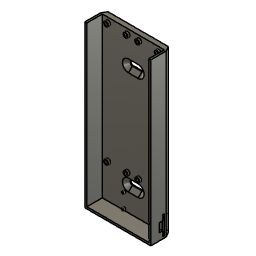
baseplate v1 (Autodesk Fusion 360 design; units mm, degrees)
Autodesk Fusion 360 part; units mm, degrees
sketch "Skizze1" plane through (0, 0, 0) normal (0, 0, 1) x (1, 0, 0)
  line L0 (0, 0) -> (62.5, 0)
  line L1 (62.5, 0) -> (62.5, 165)
  line L2 (62.5, 165) -> (0, 165)
  line L3 (0, 165) -> (0, 0)
  line L4 (31.25, 165) -> (31.25, 0) construction
  line L5 (0, 82.5) -> (62.5, 82.5) construction
  line L6 (57.5, 160) -> (5, 160) construction
  line L7 (5, 160) -> (5, 36) construction
  line L8 (5, 36) -> (57.5, 36) construction
  line L9 (57.5, 36) -> (57.5, 160) construction
  line L10 (57.5, 160) -> (5, 36) construction
  line L11 (5, 160) -> (57.5, 36) construction
  circle A0 centre (5, 36) radius 2.5
  circle A1 centre (57.5, 36) radius 2.5
  circle A2 centre (57.5, 160) radius 2.5
  circle A3 centre (5, 160) radius 2.5
  line L12 (22.1877, 17.0911) -> (63.1877, 17.0911) construction
  line L13 (63.1877, 17.0911) -> (63.1877, 2.0911) construction
  line L14 (63.1877, 2.0911) -> (22.1877, 2.0911) construction
  line L15 (22.1877, 2.0911) -> (22.1877, 17.0911) construction
  circle A4 centre (63.1877, 17.0911) radius 1.25
  circle A5 centre (63.1877, 2.0911) radius 1.25
  circle A6 centre (22.1877, 17.0911) radius 1.25
  circle A7 centre (22.1877, 2.0911) radius 1.25
  circle A8 centre (16.25, 26.2295) radius 6.25
  circle A9 centre (46.25, 26.2295) radius 6.25
  line L16 (0, 26.2295) -> (62.5, 26.2295) construction
  line L17 (37.25, 160) -> (25.25, 160) construction
  line L18 (25.25, 160) -> (25.25, 36) construction
  line L19 (25.25, 36) -> (37.25, 36) construction
  line L20 (37.25, 36) -> (37.25, 160) construction
  line L21 (37.25, 160) -> (25.25, 36) construction
  line L22 (25.25, 160) -> (37.25, 36) construction
  circle A10 centre (25.25, 160) radius 2.5
  circle A11 centre (37.25, 160) radius 2.5
  circle A12 centre (25.25, 36) radius 2.5
  circle A13 centre (37.25, 36) radius 2.5
  point P0 (31.25, 98)
  point P1 (31.25, 98)
  dimension "d1" = 62.5
  dimension "d2" = 165
  dimension "d3" = 52.5
  dimension "d4" = 124
  dimension "d5" = 5
  dimension "d6" = 5
  dimension "d7" = 5
  dimension "d8" = 5
  dimension "d9" = 5
  dimension "d10" = 41
  dimension "d11" = 15
  dimension "d13" = 2.5
  dimension "d14" = 2.5
  dimension "d15" = 2.5
  dimension "d16" = 2.5
  dimension "d17" = 12.5
  dimension "d18" = 12.5
  dimension "d19" = 15
  dimension "d20" = 15
  dimension "d25" = 12
  dimension "d26" = 5
  dimension "d27" = 5
  dimension "d28" = 5
  dimension "d29" = 5
  dimension "d30" = 124
  constraint horizontal L0
  constraint vertical L1
  constraint horizontal L2
  constraint vertical L3
  constraint coincident L0.start L3.end
  constraint midpoint L2 L4.start
  constraint midpoint L0 L4.end
  constraint midpoint L3 L5.start
  constraint midpoint L1 L5.end
  constraint horizontal L6
  constraint perpendicular L6 L7
  constraint parallel L6 L8
  constraint parallel L7 L9
  constraint coincident L10 P1
  constraint coincident L11 P1
  constraint coincident L4 P1
  constraint coincident L7.end L8.start
  constraint coincident L8.end L9.start
  constraint coincident L6.start L9.end
  constraint coincident L6.end L7.start
  constraint horizontal L12
  constraint vertical L13
  constraint horizontal L14
  constraint vertical L15
  constraint coincident L12.end L13.start
  constraint coincident L13.end L14.start
  constraint coincident L12.start L15.end
  constraint coincident L14.end L15.start
  constraint coincident L3 L16.start
  constraint coincident L1 L16.end
  constraint perpendicular L1 L16
  constraint coincident A9.centre L16
  constraint coincident A8.centre L16
  constraint horizontal L17
  constraint perpendicular L17 L18
  constraint parallel L17 L19
  constraint parallel L18 L20
  constraint coincident L21 P1
  constraint coincident L22 P1
  constraint coincident P1 P0
  constraint coincident L17.end L18.start
  constraint coincident L17.start L20.end
  constraint coincident L18.end L19.start
  constraint coincident L19.end L20.start
  measures "d1" distance of L0.start L0.end
  measures "d2" distance of L0.start L2.end
  measures "d3" distance of L7.end L8.end
  measures "d4" distance of L6.end L7.end
  measures "d5" distance of L2 L6
  measures "d6" diameter of A0
  measures "d7" diameter of A1
  measures "d8" diameter of A2
  measures "d9" diameter of A3
  measures "d10" distance of L12.start L12.end
  measures "d11" distance of L12.start L14.end
  measures "d13" diameter of A4
  measures "d14" diameter of A5
  measures "d15" diameter of A6
  measures "d16" diameter of A7
  measures "d17" diameter of A8
  measures "d18" diameter of A9
  measures "d19" distance of L4 A8.centre
  measures "d20" distance of L4 A9.centre
  measures "d25" distance of L18.end L19.end
  measures "d26" diameter of A10
  measures "d27" diameter of A11
  measures "d28" diameter of A12
  measures "d29" diameter of A13
  measures "d30" distance of L17.end L18.end
extrude "Extrusion1" add sketch "Skizze1" along normal blind 5 contours L0 L1 L2 L3 A4 A5 | L1 A5 | L1 A4 | A0 | A1 | A2 | A3 | A6 | A7 | A8 | A9 | A10 | A11 | A12 | A13 picked at (62.3027, 2.2267) picked at (62.3167, 17.1498)
extrude "Extrusion2" add sketch "Skizze1" along normal blind 7 contours L1 A5 | L1 A5 | L1 A4 | L1 A4 | A0 | A1 | A2 | A3 | A6 | A7 | A10 | A11 | A12 | A13
hole "Bohrung1" at (5, 160, 7) direction (0, 0, -1) diameter 2.6 depth 5 tip angle 180
hole "Bohrung2" at (25.25, 160, 7) direction (0, 0, -1) diameter 2.6 depth 5 tip angle 180
hole "Bohrung3" at (37.25, 160, 7) direction (0, 0, -1) diameter 2.6 depth 5 tip angle 180
hole "Bohrung4" at (57.5, 160, 7) direction (0, 0, -1) diameter 2.6 depth 5 tip angle 180
hole "Bohrung5" at (5, 36, 7) direction (0, 0, -1) diameter 2.6 depth 5 tip angle 180
hole "Bohrung6" at (25.25, 36, 7) direction (0, 0, -1) diameter 2.6 depth 5 tip angle 180
hole "Bohrung7" at (37.25, 36, 7) direction (0, 0, -1) diameter 2.6 depth 5 tip angle 180
hole "Bohrung8" at (57.5, 36, 7) direction (0, 0, -1) diameter 2.6 depth 5 tip angle 180
hole "Bohrung9" at (22.1877, 17.0911, 7) direction (0, 0, -1) diameter 1 depth 5 tip angle 180
hole "Bohrung10" at (22.1877, 2.0911, 7) direction (0, 0, -1) diameter 1 depth 5 tip angle 180
sketch "Skizze2" plane through (0, 165, 0) normal (0, 1, 0) x (-1, 0, 0)
  line L0 (-62.5, 0) -> (0, 0)
  line L1 (0, 0) -> (0, 5)
  line L2 (0, 5) -> (-62.5, 5)
  line L3 (-62.5, 5) -> (-62.5, 0)
  line L4 (0, 0) -> (2.8868, 5)
  line L5 (0, 0) -> (5.7735, 0) construction
  line L6 (2.8868, 5) -> (0, 5)
  line L7 (-62.5, 0) -> (-65.3868, 5)
  line L8 (-62.5, 0) -> (-56.7265, 0) construction
  line L9 (-65.3868, 5) -> (-62.5, 5)
  dimension "d67" = 60
  dimension "d68" = 120
  constraint horizontal L5
  constraint coincident L0.end L1.start
  constraint coincident L1.end L2.start
  constraint perpendicular L1 L6
  constraint horizontal L8
  constraint coincident L0.start L3.end
  constraint coincident L2.end L3.start
  constraint perpendicular L3 L9
  measures "d67" angle of L4 L5
  measures "d68" angle of L7 L8
extrude "Extrusion3" add sketch "Skizze2" against normal blind 165 contours L3 L7 L9 | L1 L4 L6
sketch "Skizze3" plane through (0, 0, 5) normal (0, 0, 1) x (1, 0, 0)
  circle A0 centre (37.25, 36) radius 2.5
  circle A1 centre (63.1877, 2.0911) radius 1.25
  circle A2 centre (57.5, 36) radius 2.5
  circle A3 centre (5, 160) radius 2.5
  circle A4 centre (22.1877, 17.0911) radius 1.25
  circle A5 centre (25.25, 160) radius 2.5
  circle A6 centre (25.25, 36) radius 2.5
  circle A7 centre (63.1877, 17.0911) radius 1.25
  circle A8 centre (5, 36) radius 2.5
  circle A9 centre (57.5, 160) radius 2.5
  circle A10 centre (22.1877, 2.0911) radius 1.25
  circle A11 centre (37.25, 160) radius 2.5
  line L0 (-2.8868, 0) -> (65.3868, 0)
  line L1 (65.3868, 0) -> (65.3868, 165)
  line L2 (65.3868, 165) -> (-2.8868, 165)
  line L3 (-2.8868, 165) -> (-2.8868, 0)
  line L4 (31.25, 165) -> (31.25, 0) construction
  line L5 (23.3395, 132) -> (42.0039, 132) construction
  line L6 (19.7992, 25) -> (41.2685, 25) construction
  circle A12 centre (26.25, 132) radius 2.25
  circle A13 centre (36.25, 132) radius 2.25
  line L7 (26.25, 134.25) -> (36.25, 134.25)
  line L8 (26.25, 129.75) -> (36.25, 129.75)
  line L9 (26.25, 27.25) -> (36.25, 27.25)
  circle A14 centre (26.25, 25) radius 2.25
  line L10 (26.25, 22.75) -> (36.25, 22.75)
  circle A15 centre (36.25, 25) radius 2.25
  dimension "d71" = 28
  dimension "d72" = 25
  dimension "d73" = 4.5
  dimension "d74" = 4.5
  dimension "d75" = 5
  dimension "d76" = 5
  dimension "d77" = 4.5
  dimension "d78" = 4.5
  constraint midpoint L2 L4.start
  constraint midpoint L0 L4.end
  constraint perpendicular L4 L5
  constraint perpendicular L4 L6
  constraint coincident L5 A12.centre
  constraint coincident L5 A13.centre
  constraint coincident A12 L7.start
  constraint coincident A13 L7.end
  constraint perpendicular L4 L7
  constraint coincident A12 L8.start
  constraint coincident A13 L8.end
  constraint tangent A13 L7
  constraint tangent A12 L8
  constraint tangent A13 L8
  constraint coincident L9.start A14
  constraint coincident L9.end A15
  constraint coincident L10.start A14
  constraint coincident L10.end A15
  constraint tangent L9 A15
  constraint tangent A14 L10
  constraint tangent L10 A15
  measures "d71" distance of A5.centre L5
  measures "d72" distance of L0 L6
  measures "d73" diameter of A12
  measures "d74" diameter of A13
  measures "d75" distance of L4 A12.centre
  measures "d76" distance of L4 A13.centre
  measures "d77" diameter of A14
  measures "d78" diameter of A15
extrude "Extrusion4" cut sketch "Skizze3" against normal blind 5 contours A12 | A12 A13 L7 L8 | A13 | L9 A14 L10 A15 | A14 | A15
chamfer "Fase1" distance 4 angle 45 8 edges at (38.5, 132, 5) (31.25, 129.75, 5) (24, 132, 5) (31.25, 134.25, 5) (38.5, 25, 5) (31.25, 22.75, 5) (24, 25, 5) (31.25, 27.25, 5)
sketch "Skizze4" plane through (0, 0, 0) normal (0, -1, 0) x (1, 0, 0)
  line L0 (0, 0) -> (62.5, 0)
  line L1 (62.5, 0) -> (65.3868, 5)
  line L2 (65.3868, 5) -> (-2.8868, 5)
  line L3 (-2.8868, 5) -> (0, 0)
  line L4 (65.3868, 5) -> (65.3868, 0)
  line L5 (65.3868, 0) -> (62.5, 0)
  constraint coincident L1.end L2.start
  constraint perpendicular L0 L4
  constraint coincident L0.end L1.start
  constraint perpendicular L4 L5
extrude "Extrusion5" cut sketch "Skizze4" against normal blind 20 contours L1 L4 L5
extrude "Extrusion6" add 1 faces at (20.8333, 0, 3.3333) along direction (0, -1, 0) blind 2
sketch "Skizze5" plane through (0, 0, 5) normal (0, 0, 1) x (1, 0, 0)
  arc A0 (36.25, 125.75) -> (36.25, 138.25) centre (36.25, 132) ccw
  line L0 (36.25, 125.75) -> (26.25, 125.75)
  arc A1 (26.25, 138.25) -> (26.25, 125.75) centre (26.25, 132) ccw
  line L1 (26.25, 138.25) -> (36.25, 138.25)
  circle A2 centre (63.1877, 2.0911) radius 1.25
  circle A3 centre (63.1877, 17.0911) radius 1.25
  circle A4 centre (37.25, 36) radius 2.5
  line L2 (65.3868, -2) -> (65.3868, 165)
  line L3 (65.3868, 165) -> (-2.8868, 165)
  line L4 (-2.8868, 165) -> (-2.8868, -2)
  circle A5 centre (57.5, 36) radius 2.5
  circle A6 centre (5, 160) radius 2.5
  circle A7 centre (22.1877, 17.0911) radius 1.25
  circle A8 centre (25.25, 160) radius 2.5
  circle A9 centre (25.25, 36) radius 2.5
  circle A10 centre (5, 36) radius 2.5
  circle A11 centre (57.5, 160) radius 2.5
  circle A12 centre (22.1877, 2.0911) radius 1.25
  circle A13 centre (37.25, 160) radius 2.5
  arc A14 (36.25, 18.75) -> (36.25, 31.25) centre (36.25, 25) ccw
  line L5 (36.25, 18.75) -> (26.25, 18.75)
  arc A15 (26.25, 31.25) -> (26.25, 18.75) centre (26.25, 25) ccw
  line L6 (26.25, 31.25) -> (36.25, 31.25)
  line L7 (-2.8868, 165) -> (-0.8868, 165)
  line L8 (-0.8868, 165) -> (-0.8868, 0)
  line L9 (-0.8868, 0) -> (-2.8868, 0)
  line L10 (-2.8868, 0) -> (-2.8868, 165)
  line L11 (65.3868, 165) -> (63.3868, 165)
  line L12 (63.3868, 165) -> (63.3868, 19.7779)
  line L13 (63.3868, 19.7779) -> (65.3868, 19.7779)
  line L14 (65.3868, 19.7779) -> (65.3868, 165)
  line L15 (-2.8868, -2) -> (65.3868, -2)
  line L16 (-2.8868, -2) -> (65.3868, -2)
  line L17 (65.3868, -2) -> (65.3868, 0)
  line L18 (65.3868, 0) -> (-2.8868, 0)
  line L19 (-2.8868, 0) -> (-2.8868, -2)
  dimension "d84" = 2
  dimension "d85" = 2
  dimension "d88" = 2
  constraint horizontal L7
  constraint vertical L8
  constraint horizontal L9
  constraint vertical L10
  constraint coincident L3.end L4.start
  constraint horizontal L11
  constraint vertical L12
  constraint horizontal L13
  constraint vertical L14
  constraint coincident L2.end L3.start
  constraint horizontal L16
  constraint vertical L17
  constraint horizontal L18
  constraint vertical L19
  constraint coincident L2 L17.end
  constraint coincident L4.end L15.start
  measures "d84" distance of L8 L10
  measures "d85" distance of L2.end L11.end
  measures "d88" distance of L4.end L9.end
extrude "Extrusion7" add sketch "Skizze5" along normal blind 16 contours L2 L4 L9 L15 L16 L17 L18 L19 | L2 L3 L11 L12 L13 L14 | L3 L4 L7 L8 L9 L10 L18
sketch "Skizze6" plane through (0, 19.7779, 0) normal (0, -1, 0) x (1, 0, 0)
  line L0 (63.3868, 5) -> (65.3868, 5)
  line L1 (65.3868, 5) -> (65.3868, 21)
  line L2 (65.3868, 21) -> (63.3868, 21)
  line L3 (63.3868, 21) -> (63.3868, 5)
  line L4 (63.3868, 7) -> (65.3868, 7)
  line L5 (63.3868, 8.5) -> (65.3868, 8.5)
  dimension "d91" = 2
  dimension "d92" = 3.5
  constraint coincident L3 L4.start
  constraint coincident L1 L4.end
  constraint perpendicular L1 L4
  constraint coincident L3 L5.start
  constraint coincident L1 L5.end
  constraint perpendicular L1 L5
  measures "d91" distance of L0 L4
  measures "d92" distance of L0 L5
extrude "Extrusion8" add sketch "Skizze6" along normal blind 20 contours L0 L1 L3 L4 | L1 L2 L3 L5
sketch "Skizze7" plane through (65.3868, 0, 0) normal (1, 0, 0) x (0, 0, -1)
  line L0 (-7, 0) -> (-8.5, 0)
  line L1 (-8.5, 0) -> (-8.5, 19.7779)
  line L2 (-8.5, 19.7779) -> (-7, 19.7779)
  line L3 (-7, 19.7779) -> (-7, 0)
  line L4 (-5, -2) -> (-5, 165)
  line L5 (-5, 165) -> (-21, 165)
  line L6 (-21, 165) -> (-21, -2)
  line L7 (-21, -2) -> (-5, -2)
  line L8 (-8.5, 5.3889) -> (-12, 5.3889)
  line L9 (-12, 5.3889) -> (-12, 14.3889)
  line L10 (-12, 14.3889) -> (-8.5, 14.3889)
  line L11 (-8.5, 14.3889) -> (-8.5, 5.3889)
  dimension "d95" = 3.5
  dimension "d96" = 9
  constraint horizontal L8
  constraint vertical L9
  constraint horizontal L10
  constraint vertical L11
  constraint coincident L1 L8.start
  constraint midpoint L1 L11
  measures "d95" distance of L8.start L8.end
  measures "d96" distance of L8.start L10.end
extrude "Extrusion9" cut sketch "Skizze7" against normal blind 2 contours L1 L8 L9 L10 L11
hole "Bohrung11" at (63.1877, 2.0911, 7) direction (0, 0, -1) diameter 1 depth 4.5 tip angle 180
hole "Bohrung12" at (63.1877, 17.0911, 7) direction (0, 0, -1) diameter 1 depth 4.5 tip angle 180
sketch "Skizze8" plane through (0, 0, 7) normal (0, 0, 1) x (1, 0, 0)
  circle A0 centre (63.1877, 17.0911) radius 0.5
  circle A1 centre (63.1877, 2.0911) radius 0.5
  arc A2 (63.3868, 18.3252) -> (63.3868, 15.8571) centre (63.1877, 17.0911) ccw
  line L0 (63.3868, 15.8571) -> (63.3868, 3.3252)
  arc A3 (63.3868, 3.3252) -> (63.3868, 0.8571) centre (63.1877, 2.0911) ccw
  line L1 (63.3868, 0.8571) -> (63.3868, 0)
  line L2 (63.3868, 0) -> (65.3868, 0)
  line L3 (65.3868, 0) -> (65.3868, 19.7779)
  line L4 (65.3868, 19.7779) -> (63.3868, 19.7779)
  line L5 (63.3868, 19.7779) -> (63.3868, 18.3252)
  circle A4 centre (63.1877, 17.0911) radius 1
  circle A5 centre (63.1877, 2.0911) radius 1
  dimension "d101" = 2
  dimension "d102" = 2
  constraint concentric A0 A4
  constraint concentric A1 A5
  measures "d101" diameter of A4
  measures "d102" diameter of A5
extrude "Extrusion11" cut sketch "Skizze8" along normal blind 14 contours A0 | A1 | A4 | A5
move_face "Flächen versetzen1" offset -0.1 2 faces at (64.9862, 17.062, 8.5) (64.1436, 4.584, 8.5)
extrude "Extrusion12" cut 1 faces at (64.7201, 8.3889, 12) along direction (0, 0, 1) blind 0.2
